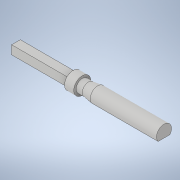
# Autodesk Inventor part: Hammer
Saved by Autodesk Inventor 2021 (Build 250183000, 183)
## iProperties
Created: 2021-03-07
Part Number: Hammer
Material: Generic
Document SubType Name: Modeling
Designer: Lukas
Density: 1 g/cm^3
Appearance: Default
Author: Lukas
Autodesk Inventor part; units mm, degrees
ref_plane "YZ Plane" through (0, 0, 0) normal (1, 0, 0) x (0, 1, 0)
ref_plane "XZ Plane" through (0, 0, 0) normal (0, 1, 0) x (-1, 0, 0)
ref_plane "XY Plane" through (0, 0, 0) normal (0, 0, 1) x (1, 0, 0)
sketch "Sketch5" plane through (0, 0, 0) normal (0, 0, 1) x (1, 0, 0)
  line L0 (-59, 0) -> (-59, 5.5)
  line L1 (-59, 5.5) -> (-53, 5.5)
  line L2 (-53, 5.5) -> (-53, 4)
  line L3 (-59, 0) -> (0, 0)
  line L4 (0, 4.85) -> (0, 0)
  line L5 (-53, 4) -> (-49, 4)
  line L6 (-49, 4) -> (-43, 4.85)
  line L7 (-43, 4.85) -> (0, 4.85)
  dimension "d83" = 5.5
  dimension "d86" = 6
  dimension "d87" = 4
  dimension "d88" = 6
  dimension "d89" = 53
  dimension "d90" = 4
  dimension "d95" = 4.85
  constraints: 16 end point, 4 horizontal, 2 vertical, 1 perpendicular
  measures "d83" distance from line of L0.start L1
  measures "d86" distance of L0.end L1.end
  measures "d87" distance between parallel lines of L3 L5
  measures "d88" horizontal distance of L5.end L6.end
  measures "d89" distance between parallel lines of L4 L2
  measures "d90" distance of L2.end L5.end
  measures "d95" distance of L4.start L3.end
revolve "Revolution1" add sketch "Sketch5" angle 360 about axis through (-59, 0, 0) along (1, 0, 0)
sketch "Sketch6" plane through (0, 0, 0) normal (1, 0, 0) x (0, 0, -1)
  circle A0 centre (0, 0) radius 4.85 projected
  circle A1 centre (0, 0) radius 4.85 projected
  line L0 (-3.8108, -3) -> (3.8108, -3)
  dimension "d96" = 3
  constraints: 2 end point, 2 point on circle, 1 horizontal
  measures "d96" distance from line of point (0, 0) L0
extrude "Extrusion5" cut sketch "Sketch6" against normal blind 53 contours L0 A0 picked at (-1.0139, -3.2592)
sketch "Sketch7" plane through (-59, 0, 0) normal (-1, 0, 0) x (0, 0, 1)
  line L0 (-2.8284, 2.8284) -> (2.8284, 2.8284)
  line L1 (2.8284, 2.8284) -> (2.8284, -2.8284)
  line L2 (2.8284, -2.8284) -> (-2.8284, -2.8284)
  line L3 (-2.8284, -2.8284) -> (-2.8284, 2.8284)
  point P0 (0, 0)
  point P1 (0, 2.8284)
  point P2 (-2.8284, 0)
  dimension "d102" = 8
  constraints: 8 end point, 2 midpoint, 2 parallel, 2 perpendicular, 1 horizontal, 1 horizontal alignment, 1 vertical alignment
  measures "d102" distance of L0.start L1.end
extrude "Extrusion6" add sketch "Sketch7" along normal blind 37
sketch "Sketch8" plane through (-96, 0, 0) normal (-1, 0, 0) x (0, 0, 1)
  circle A0 centre (0, 0) radius 1.4
  dimension "d103" = 2.8
  constraints: 1 centre point, 1 coincident
  measures "d103" diameter of A0
extrude "Extrusion7" cut sketch "Sketch8" against normal blind 10
body "Solid2"
